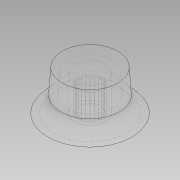
# Autodesk Inventor part: Knob
Saved by Autodesk Inventor 2016 (Build 200138000, 138)
## iProperties
Created: 2018-09-08
Part Number: Knob
Material: Generic
Document SubType Name: Modeling
Designer: Pedro Mendonça
Density: 1 g/cm^3
Appearance: Default
Author: Pedro Mendonça
Autodesk Inventor part; units mm, degrees
ref_plane "YZ Plane" through (0, 0, 0) normal (1, 0, 0) x (0, 1, 0)
ref_plane "XZ Plane" through (0, 0, 0) normal (0, 1, 0) x (-1, 0, 0)
ref_plane "XY Plane" through (0, 0, 0) normal (0, 0, 1) x (1, 0, 0)
sketch "Sketch1" plane through (0, 0, 0) normal (1, 0, 0) x (0, 1, 0)
  line L0 (0, 0) -> (0, 12.45)
  line L1 (0, 12.45) -> (8.7, 12.45)
  line L2 (8.7, 12.45) -> (9.2, 4.8665)
  line L3 (0, 0) -> (13.15, 0)
  line L4 (13.15, 0) -> (9.2, 4.8665)
  line L5 (0, -2.49) -> (0, 14.94) projected
  dimension "d5" = 12.45
  dimension "d6" = 8.7
  dimension "d7" = 7.6
  dimension "d8" = 13.15
  dimension "d10" = 9.2
  constraints: 10 end point, 1 horizontal, 1 perpendicular, 1 vertical
  measures "d5" distance of L0.start L0.end
  measures "d6" distance of L0.end L1.end
  measures "d7" distance of L1.end L2.end
  measures "d8" distance of L0.start L3.end
  measures "d10" distance from line of L2.end L0
revolve "Revolution1" add sketch "Sketch1" angle 360 about axis through (0, 0, -10) along (0, 0, 1)
sketch "Sketch2" plane through (0, 0, 0) normal (1, 0, 0) x (0, 1, 0)
  line L0 (-11.15, 0) -> (-7.2104, 4.8749)
  line L1 (-7.2173, 4.8665) -> (-6.8225, 10.8535)
  line L2 (-6.8225, 10.8535) -> (-4.8225, 10.8535)
  line L3 (-4.8225, 10.8535) -> (-4.8225, 0)
  line L4 (-11.15, 0) -> (-4.8225, 0)
  line L5 (-13.15, 0) -> (13.15, 0) projected
  line L6 (-11.15, 0) -> (-7.2173, 4.8665)
  line L7 (-6.8225, 10.8535) -> (-4.8225, 10.8535)
  line L8 (-4.8225, 0) -> (-11.15, 0)
  line L9 (0, -2.49) -> (0, 14.94) projected
  point P0 (0, 0)
  dimension "d14" = 6
  dimension "d15" = 2
  constraints: 16 end point, 2 horizontal, 2 parallel, 1 collinear
  measures "d14" distance of L1.start L1.end
  measures "d15" distance of L1.end L2.end
revolve "Revolution2" cut sketch "Sketch2" angle 360 about axis through (0, 0, -10) along (0, 0, 1)
sketch "Sketch3" plane through (0, 0, 0) normal (0, 0, -1) x (-1, 0, 0)
  circle A0 centre (0, 0) radius 3.125
  dimension "d17" = 6.25
  constraints: 1 centre point, 1 coincident
  measures "d17" diameter of A0
extrude "Extrusion1" cut sketch "Sketch3" against normal blind 8
sketch "Sketch4" plane through (0, 0, 0) normal (0, 0, -1) x (-1, 0, 0)
  circle A0 centre (0, 0) radius 3.125 projected
  circle A1 centre (0, -3.125) radius 0.485
  circle A2 centre (0.9657, -2.9721) radius 0.485
  circle A3 centre (1.8368, -2.5282) radius 0.485
  circle A4 centre (2.5282, -1.8368) radius 0.485
  circle A5 centre (2.9721, -0.9657) radius 0.485
  circle A6 centre (3.125, 0) radius 0.485
  circle A7 centre (2.9721, 0.9657) radius 0.485
  circle A8 centre (2.5282, 1.8368) radius 0.485
  circle A9 centre (1.8368, 2.5282) radius 0.485
  circle A10 centre (0.9657, 2.9721) radius 0.485
  circle A11 centre (0, 3.125) radius 0.485
  circle A12 centre (-0.9657, 2.9721) radius 0.485
  circle A13 centre (-1.8368, 2.5282) radius 0.485
  circle A14 centre (-2.5282, 1.8368) radius 0.485
  circle A15 centre (-2.9721, 0.9657) radius 0.485
  circle A16 centre (-3.125, 0) radius 0.485
  circle A17 centre (-2.9721, -0.9657) radius 0.485
  circle A18 centre (-2.5282, -1.8368) radius 0.485
  circle A19 centre (-1.8368, -2.5282) radius 0.485
  circle A20 centre (-0.9657, -2.9721) radius 0.485
  dimension "d20" = 0.97
  dimension "d23" = 360
  constraints: 20 centre point, 1 vertical alignment, 42 other
  measures "d20" diameter of A1
extrude "Extrusion2" cut sketch "Sketch4" against normal blind 8 contours A0 A6 | A0 A6 | A7 A0 | A0 A7 | A5 A0 | A0 A5 | A8 A0 | A0 A8 | A4 A0 | A0 A4 | A9 A0 | A0 A9 | A3 A0 | A0 A3 | A10 A0 | A0 A10 | A2 A0 | A0 A2 | A11 A0 | A0 A11 | A1 A0 | A0 A1 | A12 A0 | A0 A12 | A20 A0 | A0 A20 | A13 A0 | A0 A13 | A19 A0 | A0 A19 | A14 A0 | A0 A14 | A18 A0 | A0 A18 | A15 A0 | A0 A15 | A17 A0 | A0 A17 | A16 A0 | A0 A16
body "Solid1"
